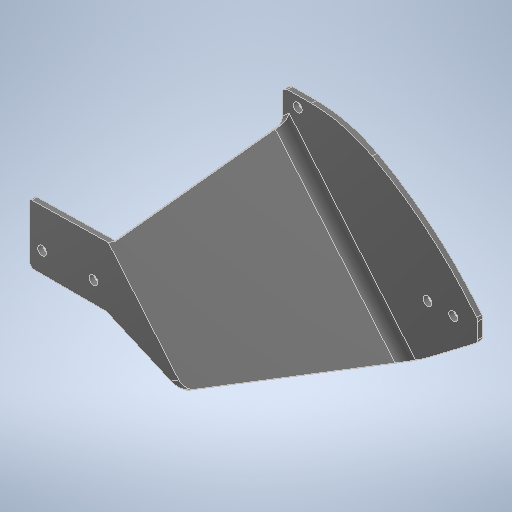
# Autodesk Inventor part: 3D_side-accessory-base-left
Saved by Autodesk Inventor 2025.1 (Build 291241020, 241B)
## iProperties
Created: 2024-09-24
Part Number: 3D_side-accessory-base-left
Material: 一般
Document SubType Name: Modeling
Designer: 8326d
Density: 1 g/cm^3
Appearance: 滑らか - 黒
Author: 8326d
Autodesk Inventor part; units mm, degrees
ref_plane "作業平面1" through (0, 0, 0) normal (0, 0, 1) x (1, 0, 0)
sketch "スケッチ1" plane through (0, 0, 0) normal (0, 0, 1) x (1, 0, 0)
  arc A0 (102.0393, 80.548) -> (61.4446, 114.5625) centre (0, 0) ccw projected
  arc A1 (102.4695, 79.3088) -> (102.0393, 80.548) centre (100.4695, 79.3088) ccw projected
  line L0 (102.4695, 73.1789) -> (102.4695, 79.3088) projected
  arc A2 (101.6775, 71.5849) -> (102.4695, 73.1789) centre (100.4695, 73.1789) ccw projected
  line L1 (60.792, 40.6002) -> (101.6775, 71.5849) projected
  circle A3 centre (92.9695, 76.5) radius 1.75 projected
  circle A4 centre (82.9695, 76.5) radius 1.75 projected
  arc A5 (61.4446, 114.5625) -> (37.812, 120.5) centre (37.812, 70.5) ccw projected
  circle A6 centre (32.5, 116.5) radius 1.75 projected
  line L2 (37.812, 120.5) -> (-37.812, 120.5) projected
  line L3 (74.6235, 51.0823) -> (26.5, 108.4337)
  line L4 (26.5, 108.4337) -> (26.5, 120.5)
  point P0 (0, 0)
  dimension "d0" = 50
  dimension "d1" = 90
  dimension "d2" = 6
  constraints: 4 end point, 2 point on line, 1 perpendicular
  measures "d0" angle of L2 L3
  measures "d1" distance from line of point (0, 0) L3
  measures "d2" distance from line of A6.centre L4
extrude "押し出し1" add sketch "スケッチ1" along normal blind 2
ref_plane "作業平面2" through (26.5, 108.4337, 0) normal (-0.7198463, -0.6040228, -0.3420201) x (0.6427876, -0.7660444, 0)
sketch "スケッチ2" plane through (26.5, 108.4337, 0) normal (-0.7198463, -0.6040228, -0.3420201) x (0.6427876, -0.7660444, 0)
  line L0 (7.112, 60.7019) -> (54.1566, 74.2031) projected
  line L1 (0, 0) -> (74.8669, 0) projected
  line L2 (0, 0) -> (7.112, 60.7019)
  line L3 (74.8669, 0) -> (48.4548, 72.5668)
  point P0 (66.0311, 30.7818)
  dimension "d6" = 70
  constraints: 4 end point, 1 point on line
  measures "d6" angle of L1 L3
extrude "押し出し2" add sketch "スケッチ2" against normal blind 2
sketch "スケッチ3" plane through (0, 0, 0) normal (1, 0, 0) x (0, 1, 0)
  line L0 (90.8485, 57.7251) -> (56.5697, 68.8745) projected
  line L1 (109.2082, 2) -> (90.8485, 57.7251) projected
  line L2 (55.3616, 68.1905) -> (56.5697, 68.8745) projected
  line L3 (51.0823, 0) -> (55.3616, 68.1905) projected
  line L4 (28.0876, 56.9615) -> (89.5, 56.9615) projected
  line L5 (89.5, 56.9615) -> (91.1001, 56.9615)
  point P0 (0, 0)
  point P1 (54.657, 56.9615)
  constraints: 2 end point, 1 horizontal, 1 point on line
extrude "押し出し3" cut sketch "スケッチ3" along normal through all
sketch "スケッチ4" plane through (46.3606, 55.8221, 56.9615) normal (0, 0, 1) x (0.7660444, 0.6427876, 0)
  line L0 (-2.1284, 0.2649) -> (-2.1284, 45.9669)
  line L1 (-23.9484, 65.3639) -> (-2.4992, 47.3658)
  arc A0 (-2.3759, 45.957) -> (-2.4992, 47.3658) centre (-3.1419, 46.5998) ccw
  line L2 (-2.3759, 45.957) -> (-41.8511, -1.0876)
  circle A1 centre (-15.2051, 38.4463) radius 1.75
  circle A2 centre (-30.526, 51.3021) radius 1.75
  line L3 (-64.8324, 18.196) -> (-25.3572, 65.2406)
  arc A3 (-23.9484, 65.3639) -> (-25.3572, 65.2406) centre (-24.5912, 64.5979) ccw
  line L4 (-2.1284, 45.9669) -> (0, 46.0522)
  line L5 (0, 46.0522) -> (0, 0)
  line L6 (0, 0) -> (-2.1284, 0.2649)
  line L7 (-39.4986, 48.3877) -> (-16.5172, 29.104)
  line L8 (-2.1284, 0.2649) -> (-16.5172, 29.104)
  line L9 (0, 46.0522) -> (-23.9635, 65.3763)
  point P0 (-71.3961, -12.9621)
extrude "押し出し4" add sketch "スケッチ4" along normal blind 2
ref_plane "作業平面3" through (66.8878, 46.8855, 2) normal (-0.1745919, 0.2698363, 0.9469456) x (-0.8395817, -0.5432335, 0)
sketch "スケッチ5" plane through (66.8878, 46.8855, 2) normal (-0.1745919, 0.2698363, 0.9469456) x (-0.8395817, -0.5432335, 0)
  line L0 (-8.6901, 0) -> (-8.7746, 0.6428) projected
  line L1 (-8.7746, 0.6428) -> (-42.6264, -1.7407) projected
  line L2 (12.3796, 0) -> (-10.1013, 0) projected
  line L3 (-10.1013, 0) -> (-17.904, 0)
  point P0 (81.6275, 2.2251)
  constraints: 2 end point, 1 horizontal, 1 point on line
extrude "押し出し5" cut sketch "スケッチ5" against normal through all
sketch "スケッチ6" plane through (26.6415, 108.265, 2) normal (-0.6689091, 0.7352575, 0.1093487) x (0.7400084, 0.6725835, 0.0043555)
  line L0 (-18.6187, -55.3752) -> (-18.61, -57.3632) projected
  line L1 (-20.4318, -62.4029) -> (-18.61, -57.3632) projected
  line L2 (-18.61, -57.3632) -> (-41.79, -55.2485) projected
  line L3 (-18.6187, -55.3752) -> (-21.1556, -62.393)
  line L4 (-22.548, -62.3739) -> (-20.4318, -62.4029) projected
  line L5 (1.4015, 0.0061) -> (-18.6187, -55.3752) projected
  point P0 (-92.5409, -5.2141)
  constraints: 2 end point, 1 collinear, 1 point on line
extrude "押し出し6" cut sketch "スケッチ6" along normal through all both and the other way through all
fillet "フィレット1" radius 5 1 edges at (51.5235, 80.7905, 2)
fillet "フィレット2" radius 2 2 edges at (28.9741, 110.3871, 2) (27.1599, 108.7366, 2)
fillet "フィレット3" radius 2 3 edges at (26.5, 120.5, 1) (-15, 67.5, 57.9615) (15, 67.5, 57.9615)
fillet "フィレット4" radius 5 1 edges at (45.1523, 55.0403, 58.9615)
